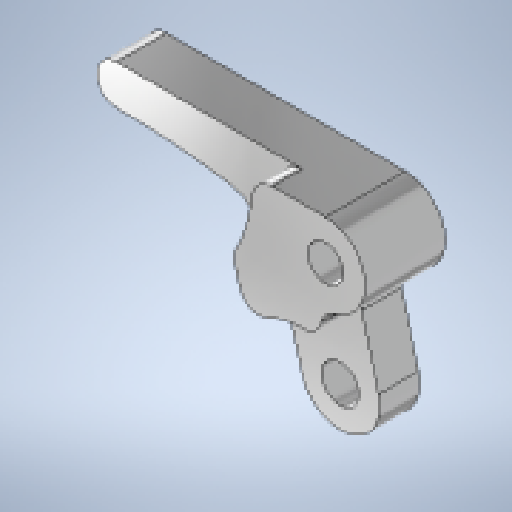
# Autodesk Inventor part: Lever
Saved by Autodesk Inventor 2023.4 (Build 274418000, 418)
## iProperties
Created: 2024-02-17
Part Number: Lever
Material: Aluminum 6061
Document SubType Name: Modeling
Designer: Nathan Cai
Density: 2.7 g/cm^3
Appearance: Aluminum - Flat
Author: Nathan Cai
Autodesk Inventor part; units mm, degrees
ref_plane "YZ Plane" through (0, 0, 0) normal (1, 0, 0) x (0, 1, 0)
ref_plane "XZ Plane" through (0, 0, 0) normal (0, 1, 0) x (-1, 0, 0)
ref_plane "XY Plane" through (0, 0, 0) normal (0, 0, 1) x (1, 0, 0)
sketch "Sketch1" plane through (0, 0, 0) normal (0, 0, 1) x (1, 0, 0)
  circle A0 centre (0, 0) radius 1.4224
  circle A1 centre (0, 0) radius 3.175
  line L0 (0, 0) -> (-19.05, 0) construction
  circle A2 centre (-2.476506, -10.833032) radius 3.175
  circle A3 centre (-2.476506, -10.833032) radius 5 construction
  circle A4 centre (-2.476506, -10.833032) radius 1.5
  line L1 (0, 0) -> (-2.476506, -10.833032) construction
  line L2 (-2.476506, -10.833032) -> (-3.938782, -10.498745) construction
  line L3 (0, 0) -> (-2.476506, -10.833032) construction
  arc A5 (-5.54332, -10.011281) -> (0.590309, -11.654782) centre (-2.476506, -10.833032) ccw
  arc A6 (-1.02973, -3.003378) -> (-19.05, 0) centre (-19.05, -55.5625) ccw
  arc A7 (-19.05, 3.175) -> (-19.05, 0) centre (-19.05, 1.5875) ccw
  line L4 (-19.05, 3.175) -> (0, 3.175)
  line L5 (-2.476506, -10.833032) -> (-4.878131, 0) construction
  line L6 (0.623234, -10.145836) -> (-1.778391, 0.687196)
  line L7 (-7.977871, -0.687196) -> (-5.576246, -11.520227)
  arc A8 (-5.576246, -11.520227) -> (0.623234, -10.145836) centre (-2.476506, -10.833032) ccw
  arc A9 (-1.778391, 0.687196) -> (-7.977871, -0.687196) centre (-4.878131, 0) ccw
  circle A10 centre (6.746875, -0.79375) radius 3.175
  circle A11 centre (6.746875, -0.79375) radius 1.5
  line L8 (7.117846, 2.359503) -> (0.370971, 3.153253)
  arc A12 (4.720646, -3.238136) -> (-0.236744, -6.266728) centre (2.761054, -5.602132) ccw
  circle A13 centre (6.746875, -0.79375) radius 5 construction
  point P0 (0.590309, -11.654782)
  point P1 (0, 3.175)
  point P2 (-7.878677, -1.134631)
  point P3 (-5.576246, -11.520227)
  point P4 (0.623234, -10.145836)
  point P5 (-0.954741, -3.028051)
  point P6 (-2.439066, 2.03263)
  point P7 (1.235308, -2.924832)
  point P8 (1.403608, -2.847896)
  point P9 (-1.424341, -1.064207)
  point P10 (-1.702423, 0.512874)
  point P11 (0.623234, -10.145836)
  point P12 (-5.576246, -11.520227)
  dimension "d24" = 3
  dimension "d0" = 2.8448
  dimension "d1" = 6.35
  dimension "d9" = 19.05
  dimension "d22" = 6.35
  dimension "d23" = 10
  dimension "d26" = 11.1125
  dimension "d29" = 3.175
  dimension "d30" = 6.35
  dimension "d31" = 6.35
  dimension "d32" = 3
  dimension "d36" = 10
  dimension "d37" = 102.5
  dimension "d38" = 4.7625
  dimension "d39" = 6.74688
  dimension "d40" = 0.79375
  constraints: 22 end point, 17 point on circle, 14 tangent, 13 centre point, 6 coincident, 2 point on line, 1 concentric, 1 horizontal, 1 parallel, 1 perpendicular, 3 other
  measures "d0" diameter of A0
  measures "d1" diameter of A1
  measures "d9" distance of L0.start L0.end
  measures "d22" diameter of A2
  measures "d23" diameter of A3
  measures "d26" distance from line of point (0, 0) L2
  measures "d29" diameter of A7
  measures "d30" diameter of A9
  measures "d31" diameter of A10
  measures "d32" diameter of A11
  measures "d36" diameter of A13
  measures "d37" angle of L0 L5
  measures "d38" distance from line of A0.centre L5
  measures "d39" horizontal distance of A0.centre A11.centre
  measures "d40" vertical distance of A0.centre A11.centre
sketch "Sketch1 outline for Extrusion1" plane through (0, 0, 0) normal (0, 0, 1) x (1, 0, 0)
  arc A0 (-19.05, 3.175) -> (-19.05, 0) centre (-19.05, 1.5875) ccw
  arc A1 (-19.05, 0) -> (-7.878677, -1.134631) centre (-19.05, -55.5625) cw
  line L0 (-7.878677, -1.134631) -> (-5.576246, -11.520227)
  arc A2 (-5.576246, -11.520227) -> (0.623234, -10.145836) centre (-2.476506, -10.833032) ccw
  line L1 (0.623234, -10.145836) -> (-0.954741, -3.028051)
  arc A3 (-0.954741, -3.028051) -> (0, 3.175) centre (0, 0) ccw
  line L2 (0, 3.175) -> (-19.05, 3.175)
  circle A4 centre (0, 0) radius 1.4224
  circle A5 centre (-2.476506, -10.833032) radius 1.5
extrude "Extrusion1" add sketch "Sketch1 outline for Extrusion1" along normal blind 3.175
fillet "Fillet1" radius 3.175 1 edges at (-7.8787, -1.1346, 1.5875)
sketch "Sketch2" plane through (0, 0, 3.175) normal (0, 0, 1) x (1, 0, 0)
  circle A0 centre (-2.476506, -10.833032) radius 1.5
  arc A1 (-0.348803, -5.761259) -> (-6.548283, -7.13565) centre (-2.476506, -10.833032) ccw
  line L0 (0, 3.175) -> (-19.05, 3.175)
  arc A2 (-19.05, 3.175) -> (-19.05, 0) centre (-19.05, 1.5875) ccw
  arc A3 (-10.006813, -0.74086) -> (-19.05, 0) centre (-19.05, -55.5625) ccw
  arc A4 (-7.423826, -3.18633) -> (-10.006813, -0.74086) centre (-10.523566, -3.873526) ccw
  line L1 (-7.423826, -3.18633) -> (-5.576246, -11.520227)
  arc A5 (-5.576246, -11.520227) -> (0.623234, -10.145836) centre (-2.476506, -10.833032) ccw
  line L2 (0.623234, -10.145836) -> (-0.954741, -3.028051)
  arc A6 (-0.954741, -3.028051) -> (0, 3.175) centre (0, 0) ccw
  circle A7 centre (0, 0) radius 1.4224
  circle A8 centre (-2.476506, -10.833032) radius 1.5
  arc A9 (-7.423826, -3.18633) -> (-10.006813, -0.74086) centre (-10.523566, -3.873526) ccw
  line L3 (0, 3.175) -> (-19.05, 3.175)
  arc A10 (-7.423826, -3.18633) -> (-5.7158, 3.175) centre (-18.4158, 3.175) ccw
  line L4 (0.623234, -10.145836) -> (-0.954741, -3.028051)
  line L5 (-7.423826, -3.18633) -> (-5.576246, -11.520227)
  point P0 (-6.548283, -7.13565)
  point P1 (-5.7158, 3.175)
  point P2 (-0.348803, -5.761259)
  dimension "d41" = 11
  dimension "d42" = 12.7
  constraints: 4 point on circle, 3 point on line, 2 centre point, 1 coincident, 1 line through centre
  measures "d41" diameter of A1
  measures "d42" radius of A10
extrude "Extrusion2" add sketch "Sketch2" along normal blind 0.79375 contours A1 L1 A10 L0 A6 L2 | A4 A3 A2 L0 A10
extrude "Extrusion3" add sketch "Sketch2" along normal blind 3.175 contours A1 L1 A10 L0 A6 L2
fillet "Fillet2" radius 1.5875 5 edges at (-6.5483, -7.1357, 4.7625) (-7.4238, -3.1863, 5.1594) (-5.7158, 3.175, 5.1594) (-0.9547, -3.0281, 3.175) (-0.3488, -5.7613, 4.7625)
body "Solid1"
